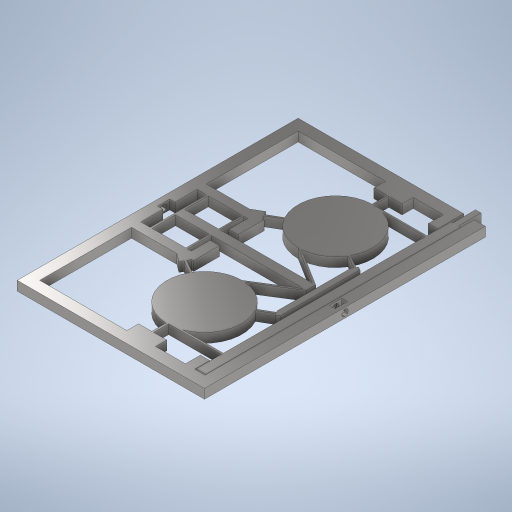
# Autodesk Inventor part: FlexBloc
Saved by Autodesk Inventor 2023 (Build 270158000, 158)
## iProperties
Created: 2023-03-17
Part Number: FlexBloc
Material: Steel, Mild
Document SubType Name: Modeling
Designer: Nathann
Density: 7.85 g/cm^3
Appearance: Semi-Polished
Mass: 385.209 g
Surface Area: 310.59 cm^2
Volume: 49.0711 cm^3
Author: Nathann
Autodesk Inventor part; units mm, degrees
ref_plane "YZ Plane" through (0, 0, 0) normal (1, 0, 0) x (0, 1, 0)
ref_plane "XZ Plane" through (0, 0, 0) normal (0, 1, 0) x (-1, 0, 0)
ref_plane "XY Plane" through (0, 0, 0) normal (0, 0, 1) x (1, 0, 0)
sketch "Sketch1" plane through (0, 0, 0) normal (0, 1, 0) x (-1, 0, 0)
  line L0 (0, 0) -> (100, 0)
  line L1 (100, 0) -> (100, 150)
  line L2 (100, 150) -> (0, 150)
  line L3 (0, 150) -> (0, 0)
  dimension "d0" = 150
  dimension "d1" = 100
  constraints: 8 end point, 2 parallel, 1 horizontal, 1 perpendicular
  measures "d0" distance of L2.end L0.start
  measures "d1" distance of L0.start L0.end
extrude "Extrusion1" add sketch "Sketch1" along normal blind 5
sketch "Sketch6" plane through (0, 5, 0) normal (0, 1, 0) x (1, 0, 0)
  line L0 (0, 0) -> (-5, 0)
  line L1 (-100, 0) -> (-100, -150) projected
  line L2 (-6, -143.6874) -> (-6, -6)
  line L3 (0, -150) -> (0, 0) projected
  line L4 (-100, -150) -> (0, -150) projected
  line L5 (0, 0) -> (-100, 0) projected
  line L6 (-11.5, -143.6874) -> (-16.5, -143.6874)
  line L7 (-16.5, -143.6874) -> (-16.5, -135.6874)
  line L8 (-16.5, -135.6874) -> (-11.5, -135.6874)
  line L9 (-11.5, -135.6874) -> (-11.5, -143.6874)
  line L10 (-11.25, -143) -> (-6.25, -143)
  line L11 (-6.25, -143) -> (-6.25, -7)
  line L12 (-6.25, -7) -> (-11.25, -7)
  line L13 (-11.5, -6) -> (-16.5, -6)
  line L14 (-16.5, -6) -> (-16.5, -14)
  line L15 (-16.5, -14) -> (-11.5, -14)
  line L16 (-11.5, -14) -> (-11.5, -6)
  line L17 (-11.5, -6) -> (-11.5, 0)
  line L18 (-6, 0) -> (-6, -6)
  line L19 (-100, 0) -> (-100, -150)
  line L20 (-100, -150) -> (0, -150)
  line L21 (0, -150) -> (0, 0)
  line L22 (0, 0) -> (-6, 0)
  line L23 (-11.5, 0) -> (-100, 0)
  line L24 (-10.25, -7) -> (-7.25, -7)
  line L25 (-7.25, -7) -> (-7.25, 13)
  line L26 (-7.25, 13) -> (-10.25, 13)
  line L27 (-10.25, 13) -> (-10.25, -7)
  line L28 (-11.25, -129.1874) -> (-33.5419, -129.1874)
  line L29 (-40, -20) -> (-11.25, -20)
  line L30 (-11.25, -21) -> (-33.755, -21)
  line L31 (-40, -90) -> (-19.9958, -77.5)
  line L32 (-19.9958, -72.5) -> (-40, -60)
  line L33 (-38.2375, -59.9222) -> (-18.1087, -72.5)
  line L34 (-18.1087, -77.5) -> (-38.2375, -90.0778)
  arc A0 (-40.5, -20.0063) -> (-40, -60) centre (-40, -40) ccw
  line L35 (-11.25, -129.6874) -> (-11.25, -143)
  line L36 (-11.25, -7) -> (-11.25, -20)
  line L37 (-11.25, -21) -> (-11.25, -128.6874)
  line L38 (-19.9958, -72.5) -> (-89, -72.5)
  line L39 (-89, -72.5) -> (-89, -77.5)
  line L40 (-89, -77.5) -> (-19.9958, -77.5)
  line L41 (-94, -55) -> (-69, -55)
  line L42 (-69, -55) -> (-69, -60)
  line L43 (-69, -60) -> (-94, -60)
  line L44 (-94, -60) -> (-94, -55)
  line L45 (-94, -90) -> (-69, -90)
  line L46 (-69, -90) -> (-69, -95)
  line L47 (-69, -95) -> (-94, -95)
  line L48 (-94, -95) -> (-94, -90)
  line L49 (-40, -90) -> (-40, -77.5)
  line L50 (-40, -72.5) -> (-40, -60)
  line L51 (-89, -77.5) -> (-88, -77.5)
  line L52 (-88, -77.5) -> (-88, -90)
  line L53 (-88, -90) -> (-89, -90)
  line L54 (-89, -90) -> (-89, -77.5)
  line L55 (-89, -72.5) -> (-88, -72.5)
  line L56 (-88, -72.5) -> (-88, -60)
  line L57 (-88, -60) -> (-89, -60)
  line L58 (-89, -60) -> (-89, -72.5)
  line L59 (-69, -90) -> (-70, -90)
  line L60 (-70, -90) -> (-70, -77.5)
  line L61 (-70, -77.5) -> (-69, -77.5)
  line L62 (-69, -77.5) -> (-69, -90)
  line L63 (-69, -60) -> (-70, -60)
  line L64 (-70, -60) -> (-70, -72.5)
  line L65 (-70, -72.5) -> (-69, -72.5)
  line L66 (-69, -72.5) -> (-69, -60)
  line L67 (-69, -95) -> (-67, -95)
  line L68 (-67, -95) -> (-67, -90)
  line L69 (-67, -90) -> (-69, -90)
  line L70 (-69, -90) -> (-69, -95)
  line L71 (-67, -95) -> (-63.6713, -95)
  line L72 (-62, -95) -> (-62, -80)
  line L73 (-62, -80) -> (-67, -80)
  line L74 (-67, -80) -> (-67, -95)
  line L75 (-69, -55) -> (-67, -55)
  line L76 (-67, -55) -> (-67, -60)
  line L77 (-67, -60) -> (-69, -60)
  line L78 (-69, -60) -> (-69, -55)
  line L79 (-67, -55) -> (-62, -55)
  line L80 (-62, -55) -> (-62, -70)
  line L81 (-62, -70) -> (-67, -70)
  line L82 (-67, -70) -> (-67, -55)
  line L83 (-40, -110) -> (-16.022, -96.1563)
  line L84 (-40, -110) -> (-63.978, -96.1563)
  line L85 (-40, -110) -> (-40, -137.6874)
  line L86 (-20, -110) -> (-27.0715, -110)
  line L87 (-16.5013, -94.701) -> (-15.0013, -97.299)
  line L88 (-15.0013, -97.299) -> (-13.25, -96.2879)
  line L89 (-13.25, -96.2879) -> (-13.25, -53.7026)
  line L90 (-22.4349, -100.4361) -> (-15.5013, -96.433)
  line L91 (-22.9349, -99.5701) -> (-16.0013, -95.567)
  line L92 (-40, -40) -> (-15.7513, -54)
  line L93 (-40, -40) -> (-40, -12)
  line L94 (-40, -40) -> (-64.2487, -54)
  line L95 (-20, -40) -> (-22.9877, -40)
  line L96 (-16.5013, -55.299) -> (-15.0013, -52.701)
  line L97 (-16.5013, -55.299) -> (-16.5013, -71.9669)
  line L98 (-15.0013, -52.701) -> (-13.25, -53.7026)
  line L99 (-16.0013, -54.433) -> (-22.9349, -50.4299)
  line L100 (-15.5013, -53.567) -> (-22.4349, -49.5639)
  line L101 (-18.1087, -77.5) -> (-18.1087, -72.5)
  line L102 (-16.5013, -94.701) -> (-16.5013, -72.5)
  line L103 (-16.5013, -72.5) -> (-16.5013, -71.9669)
  line L104 (-40.5, -137.6874) -> (-40.5, -129.9937)
  line L105 (-39.5, -137.6874) -> (-39.5, -129.6874)
  arc A1 (-32.8738, -128.6874) -> (-22.4349, -100.4361) centre (-40, -110) ccw
  arc A2 (-22.6795, -100) -> (-38.2375, -90.0778) centre (-40, -110) ccw
  line L106 (-43.25, -138.6874) -> (-43.25, -142)
  line L107 (-36.75, -138.6874) -> (-36.75, -142)
  line L108 (-40.5, -20.0063) -> (-40.5, -12)
  arc A3 (-38.2375, -59.9222) -> (-22.9349, -50.4299) centre (-40, -40) ccw
  arc A4 (-22.6795, -50) -> (-33.755, -21) centre (-40, -40) ccw
  line L109 (-39.5, -12) -> (-39.5, -20)
  line L110 (-43.25, -11) -> (-43.25, -8)
  line L111 (-36.75, -11) -> (-36.75, -8)
  line L112 (-62.9889, -93.818) -> (-65.4889, -98.1481)
  line L113 (-64.4987, -96.433) -> (-57.5651, -100.4361)
  line L114 (-63.9987, -95.567) -> (-57.0651, -99.5701)
  arc A5 (-40, -90) -> (-57.0651, -99.5701) centre (-40, -110) ccw
  arc A6 (-57.3205, -100) -> (-40.3935, -129.9961) centre (-40, -110) ccw
  line L115 (-65.4889, -98.1481) -> (-69.708, -95)
  line L116 (-62.9889, -93.818) -> (-62, -93.818)
  line L117 (-65.4987, -51.8349) -> (-62.9987, -56.1651)
  line L118 (-63.9987, -54.433) -> (-57.0651, -50.4299)
  line L119 (-64.4987, -53.567) -> (-57.5651, -49.5639)
  line L120 (-65.4987, -51.8349) -> (-70.9808, -55)
  line L121 (-62.9987, -56.1651) -> (-62, -56.1651)
  line L122 (-37.5, -137.6874) -> (-32.5, -137.6874)
  line L123 (-32.5, -137.6874) -> (-32.5, -143.6874)
  line L124 (-36.75, -142) -> (-36.75, -138.6874)
  line L125 (-42.5, -137.6874) -> (-47.5, -137.6874)
  line L126 (-47.5, -137.6874) -> (-47.5, -144)
  line L127 (-43.25, -142) -> (-43.25, -138.6874)
  line L128 (-37.5, -12) -> (-32.5, -12)
  line L129 (-32.5, -12) -> (-32.5, -6)
  line L130 (-36.75, -8) -> (-36.75, -11)
  line L131 (-42.5, -12) -> (-47.5, -12)
  line L132 (-47.5, -12) -> (-47.5, -6)
  line L133 (-43.25, -8) -> (-43.25, -11)
  line L134 (-43.25, -138.6874) -> (-36.75, -138.6874)
  line L135 (-36.75, -11) -> (-43.25, -11)
  line L136 (-47.5, -6) -> (-94, -6)
  line L137 (-11.5, -6) -> (-32.5, -6)
  line L138 (-36.75, -8) -> (-43.25, -8)
  line L139 (-32.5, -143.6874) -> (-6, -143.6874)
  line L140 (-94, -144) -> (-47.5, -144)
  line L141 (-43.25, -142) -> (-36.75, -142)
  line L142 (-42.5, -137.6874) -> (-40.5, -137.6874)
  line L143 (-40, -137.6874) -> (-37.5, -137.6874)
  line L144 (-37.5, -12) -> (-39.5, -12)
  line L145 (-40.5, -12) -> (-42.5, -12)
  line L146 (-39.5, -129.6874) -> (-11.25, -129.6874)
  line L147 (-43.25, -6) -> (-36.75, -6)
  line L148 (-36.75, -6) -> (-36.75, -3)
  line L149 (-36.75, -3) -> (-43.25, -3)
  line L150 (-43.25, -3) -> (-43.25, -6)
  line L151 (-43.25, -144) -> (-36.75, -144)
  line L152 (-36.75, -144) -> (-36.75, -147)
  line L153 (-36.75, -147) -> (-43.25, -147)
  line L154 (-43.25, -147) -> (-43.25, -144)
  line L155 (-40, -150) -> (-40, -149.019)
  line L156 (-40, 0) -> (-40, -1.9202)
  line L157 (-94, -78.25) -> (-96.8747, -78.25)
  line L158 (-96.8747, -78.25) -> (-96.8747, -71.75)
  line L159 (-96.8747, -71.75) -> (-94, -71.75)
  line L160 (-94, -71.75) -> (-94, -72.5)
  line L161 (-94, -77.5) -> (-94, -78.25)
  line L162 (-94, -6) -> (-94, -71.75)
  line L163 (-94, -78.25) -> (-94, -144)
  line L164 (-47.5, -137.6874) -> (-94, -137.6874)
  line L165 (-70.75, -95) -> (-70.75, -137.6874)
  line L166 (-71.7543, -55) -> (-71.7543, -6)
  line L167 (-47.5, -12) -> (-71.7543, -12)
  line L168 (-11.25, -128.6874) -> (-32.8738, -128.6874)
  point P0 (-89, -75)
  point P1 (-14, -14)
  point P2 (-69, -92.5)
  point P3 (-15.7513, -96)
  point P4 (-15.7513, -54)
  point P5 (-64.2389, -95.983)
  point P6 (-88, -77.5)
  point P7 (-69, -72.5)
  point P8 (-63.6714, -55)
  point P9 (-10.25, 0)
  point P10 (-7.25, 0)
  point P11 (-36.75, -145.5)
  point P12 (-12, -136)
  point P13 (-11.5, -143)
  point P14 (-40, -129.9961)
  point P15 (-39, -138)
  point P16 (-64.2487, -96)
  point P17 (-16.5013, -72.3253)
  point P18 (-16.5013, -77.6747)
  dimension "d266" = 6.5
  dimension "d89" = 6
  dimension "d94" = 136
  dimension "d96" = 8
  dimension "d97" = 5
  dimension "d98" = 5.5
  dimension "d100" = 5
  dimension "d101" = 5.5
  dimension "d103" = 3
  dimension "d104" = 20
  dimension "d106" = 0.25
  dimension "d112" = 40
  dimension "d113" = 40
  dimension "d117" = 1
  dimension "d118" = 1
  dimension "d119" = 1
  dimension "d124" = 25
  dimension "d125" = 30
  dimension "d126" = 5
  dimension "d127" = 5
  dimension "d128" = 40
  dimension "d129" = 55
  dimension "d131" = 20
  dimension "d134" = 1
  dimension "d135" = 1
  dimension "d138" = 58
  dimension "d139" = 58
  dimension "d140" = 58
  dimension "d141" = 58
  dimension "d142" = 15
  dimension "d145" = 8
  dimension "d150" = 1
  dimension "d151" = 1
  dimension "d153" = 2
  dimension "d154" = 2
  dimension "d155" = 5
  dimension "d156" = 5
  dimension "d157" = 15
  dimension "d158" = 15
  dimension "d159" = 40
  dimension "d160" = 40
  dimension "d161" = 0
  dimension "d162" = 5
  dimension "d167" = 360
  dimension "d169" = 30
  dimension "d171" = 2
  dimension "d172" = 5
  dimension "d173" = 3
  dimension "d175" = 1.5
  dimension "d176" = 1
  dimension "d177" = 0.5
  dimension "d178" = 0.5
  dimension "d179" = 28
  dimension "d180" = 0
  dimension "d181" = 28
  dimension "d184" = 360
  dimension "d186" = 30
  dimension "d187" = 3
  dimension "d188" = 1.5
  dimension "d189" = 1
  dimension "d190" = 0.5
  dimension "d192" = 0
  dimension "d193" = 0
  dimension "d194" = 5
  dimension "d195" = 2.5
  constraints: 331 end point, 65 parallel, 58 perpendicular, 43 point on line, 37 horizontal, 22 point on circle, 9 midpoint, 8 vertical, 7 centre point, 5 coincident, 16 other
  measures "d89" distance between parallel lines of L3 L2
  measures "d94" distance of L10.end L11.end
  measures "d96" distance of L8.end L6.start
  measures "d97" distance of L7.end L8.end
  measures "d98" distance between parallel lines of L2 L9
  measures "d100" distance of L14.end L15.end
  measures "d101" distance between parallel lines of L2 L16
  measures "d103" distance of L25.end L26.end
  measures "d104" distance of L26.end L24.start
  measures "d106" distance between parallel lines of L2 L11
  measures "d112" distance from line of L4 L83.start
  measures "d113" distance from line of L5 L92.start
  measures "d117" distance between parallel lines of L30 L29
  measures "d118" distance between parallel lines of L31 L34
  measures "d119" distance between parallel lines of L32 L33
  measures "d124" distance of L45.start L45.end
  measures "d125" distance between parallel lines of L43 L45
  measures "d126" distance between parallel lines of L41 L43
  measures "d127" distance between parallel lines of L45 L47
  measures "d128" distance between parallel lines of L41 L47
  measures "d129" distance between parallel lines of L4 L47
  measures "d131" radius of A0
  measures "d134" distance between parallel lines of L52 L54
  measures "d135" distance between parallel lines of L58 L56
  measures "d138" angle of L31 L49
  measures "d139" angle of L50 L32
  measures "d140" angle of L49 L34
  measures "d141" angle of L50 L33
  measures "d142" distance from line of L45 point (-89, -75)
  measures "d145" distance of L13.end L14.end
  measures "d150" distance between parallel lines of L62 L60
  measures "d151" distance between parallel lines of L66 L64
  measures "d153" distance from line of point (-69, -92.5) L74
  measures "d154" distance between parallel lines of L42 L82
  measures "d155" distance of L72.end L73.end
  measures "d156" distance of L80.end L81.end
  measures "d157" distance of L72.start L72.end
  measures "d158" distance of L79.end L80.end
  measures "d159" distance from line of L83.start L21
  measures "d160" distance from line of L21 L92.start
  measures "d161" distance between parallel lines of L49 L50
  measures "d162" distance between parallel lines of L38 L40
  measures "d169" angle of L83 L86
  measures "d171" distance between parallel lines of L89 L37
  measures "d172" distance between parallel lines of L11 L37
  measures "d173" distance of L87.start L87.end
  measures "d175" distance between parallel lines of L83 L88
  measures "d176" distance between parallel lines of L90 L91
  measures "d177" distance between parallel lines of L90 L83
  measures "d178" distance between parallel lines of L91 L83
  measures "d179" distance from line of L84.start L87
  measures "d180" horizontal distance of L31.start L84.start
  measures "d181" distance of L92.start L92.end
  measures "d186" angle of L92 L95
  measures "d187" distance of L96.start L96.end
  measures "d188" distance from line of L96.end L92
  measures "d189" distance between parallel lines of L100 L99
  measures "d190" distance between parallel lines of L92 L99
  measures "d192" vertical distance of L34.start L31.end
  measures "d193" vertical distance of L33.end L32.start
  measures "d194" distance of L125.start L122.start
  measures "d195" distance from line of L85 L122.start
extrude "Extrusion6" cut sketch "Sketch6" against normal blind 10 contours L18 L2 L139 L9 L8 L7 L123 L122 L143 L105 L146 L35 L10 L11 L12 L25 L5 | L27 L12 L36 L29 L109 L144 L128 L129 L137 L14 L15 L16 L17 L5 | A4 L30 L37 L168 A1 L90 L87 L88 L89 L98 L96 L100 | L119 L117 L120 L41 L166 L167 L131 L145 L108 A0 | A0 L50 L38 L66 L77 L82 L81 L80 L79 L117 L118 | L96 L97 L103 L102 L87 L91 A2 L34 L101 L33 A3 L99 | L32 L38 L50 | L79 L80 L121 L117 | A6 L104 L142 L125 L164 L165 L47 L115 L112 L113 | L167 L166 L136 L132 | L41 L162 L136 L166 | L38 L56 L43 L64 | L112 L116 L72 L73 L74 L69 L62 L40 L49 A5 L114 | L43 L58 L39 L54 L45 L163 L157 L158 L159 L162 | L49 L40 L31 | L165 L164 L163 L47 | L126 L140 L163 L164 | L40 L60 L45 L52
sketch "Sketch7" plane through (0, 5, 0) normal (0, 1, 0) x (1, 0, 0)
  line L0 (-10.25, -7) -> (-10.25, 0) projected
  line L1 (-10.25, 0) -> (-7.25, 0)
  line L2 (-7.25, 0) -> (-7.25, 5)
  line L3 (-7.25, 5) -> (-10.25, 5)
  line L4 (-10.25, 5) -> (-10.25, 0)
  point P0 (0, 0)
  dimension "d253" = 5
  constraints: 8 end point, 2 parallel, 1 horizontal, 1 perpendicular
  measures "d253" distance of L1.end L2.end
extrude "Extrusion7" add sketch "Sketch7" against normal blind 5
sketch "Sketch9" plane through (0, 5, 0) normal (0, 1, 0) x (1, 0, 0)
  line L0 (-5, -78.25) -> (-2, -78.25)
  line L1 (-2, -78.25) -> (-2, -71.75)
  line L2 (-2, -71.75) -> (-5, -71.75)
  line L3 (-5, -71.75) -> (-5, -78.25)
  line L4 (0, -150) -> (0, 0) projected
  line L5 (-6, 0) -> (-6, -143.6874) projected
  line L6 (0, 0) -> (-6, 0) projected
  line L7 (-100, -150) -> (0, -150) projected
  line L8 (-16.5013, -94.701) -> (-16.5013, -77.6747) projected
  line L9 (-16.5013, -79.3479) -> (-17.3228, -79.3479)
  line L10 (-17.3228, -79.3479) -> (-17.3228, -70.2922)
  line L11 (-17.3228, -70.2922) -> (-16.5013, -70.2922)
  line L12 (-16.5013, -70.2922) -> (-16.5013, -79.3479)
  point P0 (-7.25, 0)
  dimension "d265" = 3
  dimension "d266" = 6.5
  dimension "d267" = 6
  dimension "d268" = 1
  dimension "d269" = 150
  dimension "d270" = 71.75
  constraints: 16 end point, 4 parallel, 2 horizontal, 2 perpendicular, 1 point on line
  measures "d265" distance between parallel lines of L3 L1
  measures "d266" distance of L0.end L1.end
  measures "d267" distance between parallel lines of L4 L5
  measures "d268" distance between parallel lines of L5 L3
  measures "d269" distance between parallel lines of L6 L7
  measures "d270" distance between parallel lines of L0 L7
extrude "Extrusion9" cut sketch "Sketch9" against normal blind 10
sketch "Sketch10" plane through (0, 0, 150) normal (1, 0, 0) x (0, 0, -1)
  circle A0 centre (75, 2.5) radius 1.75
  line L0 (0, 0) -> (0, 5) projected
  line L1 (0, 0) -> (150, 0) projected
  line L2 (0, 5) -> (150, 5) projected
  dimension "d273" = 75
  dimension "d274" = 3.5
  dimension "d275" = 2.5
  dimension "d276" = 5
  constraints: 1 centre point
  measures "d273" distance from line of L0 A0.centre
  measures "d274" diameter of A0
  measures "d275" distance from line of L1 A0.centre
  measures "d276" distance between parallel lines of L2 L1
extrude "Extrusion10" cut sketch "Sketch10" against normal blind 12
sketch "Sketch11" plane through (-100, 0, 0) normal (-1, 0, 0) x (0, 0, 1)
  circle A0 centre (75, 2.5) radius 1.75
  line L0 (0, 5) -> (150, 5) projected
  line L1 (0, 0) -> (150, 0) projected
  line L2 (150, 0) -> (150, 5) projected
  dimension "d279" = 5
  dimension "d280" = 2.5
  dimension "d281" = 3.5
  dimension "d282" = 75
  constraints: 1 centre point
  measures "d279" distance between parallel lines of L0 L1
  measures "d280" distance from line of L0 A0.centre
  measures "d281" diameter of A0
  measures "d282" distance from line of L2 A0.centre
extrude "Extrusion11" cut sketch "Sketch11" against normal blind 8
equation "\"d2\" = woodThickness"
equation "\"d96\" = d145"
equation "\"d98\" = d101"
equation "\"d113\" = d112"
equation "\"d117\" = bladeThickness"
equation "\"d118\" = d116"
equation "\"d119\" = bladeThickness"
equation "\"d127\" = d126"
equation "\"d134\" = bladeThickness"
equation "\"d142\" = 0.5 * d125"
equation "\"bladeThickness\" = 1"
equation "\"woodThickness\" = 5"
equation "\"bladeLenghtFlexRatio\" = 0.05"
equation "\"colRadius\" = 3"
equation "\"d14\" = bladeThickness"
equation "\"d16\" = d14"
equation "\"d19\" = d16"
equation "\"d116\" = bladeThickness"
equation "\"d121\" = d120"
equation "\"M3Hole\" = 3"
equation "\"d120\" = 65deg"
body "Solid1"
